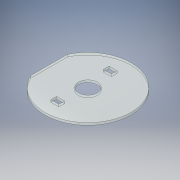
# Autodesk Inventor part: Frame 2
Saved by Autodesk Inventor 2017 (Build 210142000, 142)
## iProperties
Created: 2017-05-26
Part Number: Frame 2
Material: Glass
Document SubType Name: Modeling
Designer: anirudh
Density: 2.18 g/cm^3
Appearance: Clear
Author: anirudh
Autodesk Inventor part; units mm, degrees
ref_plane "YZ Plane" through (0, 0, 0) normal (1, 0, 0) x (0, 1, 0)
ref_plane "XZ Plane" through (0, 0, 0) normal (0, 1, 0) x (-1, 0, 0)
ref_plane "XY Plane" through (0, 0, 0) normal (0, 0, 1) x (1, 0, 0)
sketch "Sketch1" plane through (0, 0, 0) normal (0, 1, 0) x (-1, 0, 0)
  circle A0 centre (0, 0) radius 240
  circle A1 centre (0, 0) radius 52.5
  line L0 (0, 198.75) -> (70, 198.75)
  line L1 (0, -93.75) -> (70, -93.75)
  line L2 (70, 198.75) -> (-70, 198.75)
  line L3 (-70, 198.75) -> (-70, 93.75)
  line L4 (-70, 93.75) -> (70, 93.75)
  line L5 (70, 93.75) -> (70, 198.75)
  line L6 (70, -93.75) -> (-70, -93.75)
  line L7 (-70, -93.75) -> (-70, -198.75)
  line L8 (-70, -198.75) -> (70, -198.75)
  line L9 (70, -198.75) -> (70, -93.75)
  constraints: 20 end point, 4 horizontal, 4 parallel, 2 centre point, 2 coincident, 2 perpendicular
extrude "Extrusion1" add sketch "Sketch1" along normal blind 12.7
sketch "Sketch3" plane through (0, 12.7, 0) normal (0, 1, 0) x (1, 0, 0)
  circle A0 centre (0, 0) radius 240 projected
  line L0 (-217.2, 102.0988) -> (-217.2, -102.0988)
  arc A1 (-217.2, 102.0988) -> (-217.2, -102.0988) centre (0, 0) ccw
  constraints: 4 point on circle, 2 end point, 1 centre point
extrude "Extrusion2" cut sketch "Sketch3" against normal blind 12.7 contours L0 A0 picked at (-219.9077, 27.547)
sketch "Sketch5" plane through (0, 12.7, 0) normal (0, 1, 0) x (1, 0, 0)
  line L0 (70, 198.75) -> (-70, 198.75) projected
  line L1 (-70, 93.75) -> (70, 93.75) projected
  line L2 (0, 146.25) -> (0, 162.125)
  line L3 (0, 162.125) -> (-44.45, 162.125)
  line L4 (-44.45, 162.125) -> (-44.45, 130.375)
  line L5 (-44.45, 130.375) -> (0, 130.375)
  line L6 (0, 146.25) -> (0, 130.375)
  line L7 (70, 198.75) -> (-70, 198.75)
  line L8 (-70, 198.75) -> (-70, 93.75)
  line L9 (-70, 93.75) -> (70, 93.75)
  line L10 (70, 93.75) -> (70, 198.75)
  line L11 (70, -198.75) -> (70, -93.75) projected
  line L12 (-70, -198.75) -> (70, -198.75) projected
  line L13 (70, -93.75) -> (-70, -93.75)
  line L14 (-70, -93.75) -> (-70, -198.75)
  line L15 (-70, -198.75) -> (70, -198.75)
  line L16 (70, -198.75) -> (70, -93.75)
  line L17 (0, -146.25) -> (0, -130.375)
  line L18 (0, -130.375) -> (-44.45, -130.375)
  line L19 (-44.45, -130.375) -> (-44.45, -162.125)
  line L20 (-44.45, -162.125) -> (0, -162.125)
  line L21 (0, -146.25) -> (0, -162.125)
  point P0 (0, 0)
  dimension "d31" = 15.875
  dimension "d32" = 44.45
  dimension "d33" = 31.75
  dimension "d34" = 15.875
  dimension "d35" = 44.45
  dimension "d36" = 31.75
  constraints: 36 end point, 7 perpendicular, 4 parallel, 2 horizontal
  measures "d31" distance of L2.start L2.end
  measures "d32" distance of L2.end L3.end
  measures "d33" distance of L3.end L4.end
  measures "d34" distance of L17.start L17.end
  measures "d35" distance of L17.end L18.end
  measures "d36" distance of L18.end L19.end
extrude "Extrusion3" add sketch "Sketch5" against normal blind 12.7
body "Solid1"
